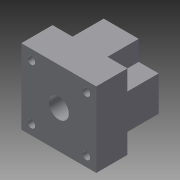
# Autodesk Inventor part: dop_krepl_k_sponke_ne_motora
Saved by Autodesk Inventor 2015 (Build 190159000, 159)
## iProperties
Created: 2016-05-14
Part Number: dop_krepl_k_sponke_ne_motora
Material: Generic
Document SubType Name: Modeling
Designer: Andreas
Density: 1 g/cm^3
Appearance: Default
Author: Andreas
Autodesk Inventor part; units mm, degrees
ref_plane "YZ Plane" through (0, 0, 0) normal (1, 0, 0) x (0, 1, 0)
ref_plane "XZ Plane" through (0, 0, 0) normal (0, 1, 0) x (-1, 0, 0)
ref_plane "XY Plane" through (0, 0, 0) normal (0, 0, 1) x (1, 0, 0)
sketch "Sketch1" plane through (0, 0, 0) normal (0, 1, 0) x (-1, 0, 0)
  line L0 (0, 0) -> (0, -30)
  line L1 (0, -30) -> (30, -30)
  line L2 (30, -30) -> (30, 0)
  line L3 (30, 0) -> (0, 0)
  point P0 (0, -15)
  point P1 (15, 0)
  dimension "d0" = 30
  dimension "d1" = 30
  constraints: 8 end point, 2 midpoint, 2 perpendicular, 1 horizontal, 1 vertical
  measures "d0" distance of L0.start L0.end
  measures "d1" distance of L0.end L1.end
extrude "Extrusion2" add sketch "Sketch1" along normal blind 25
sketch "Sketch5" plane through (0, 25, 0) normal (0, 1, 0) x (1, 0, 0)
  line L0 (0, 0) -> (-8, 0)
  line L1 (-8, 0) -> (-8, 8)
  line L2 (-8, 8) -> (0, 8)
  line L3 (0, 8) -> (0, 0)
  line L4 (0, 30) -> (-8, 30)
  line L5 (-8, 30) -> (-8, 22)
  line L6 (-8, 22) -> (0, 22)
  line L7 (0, 22) -> (0, 30)
  line L8 (-30, 30) -> (-22, 30)
  line L9 (-22, 30) -> (-22, 22)
  line L10 (-22, 22) -> (-30, 22)
  line L11 (-30, 22) -> (-30, 30)
  line L12 (-30, 0) -> (-22, 0)
  line L13 (-22, 0) -> (-22, 8)
  line L14 (-22, 8) -> (-30, 8)
  line L15 (-30, 8) -> (-30, 0)
  dimension "d22" = 8
  dimension "d23" = 8
  dimension "d24" = 8
  dimension "d25" = 8
  dimension "d26" = 8
  dimension "d27" = 8
  dimension "d28" = 8
  dimension "d29" = 8
  constraints: 32 end point, 8 parallel, 4 horizontal, 4 perpendicular
  measures "d22" distance of L1.end L2.end
  measures "d23" distance of L0.end L1.end
  measures "d24" distance of L6.end L5.end
  measures "d25" distance of L5.end L4.end
  measures "d26" distance of L9.end L10.end
  measures "d27" distance of L8.end L9.end
  measures "d28" distance of L14.end L13.end
  measures "d29" distance of L13.end L12.end
extrude "Extrusion6" cut sketch "Sketch5" against normal blind 12.5
sketch "Sketch6" plane through (0, 12.5, 0) normal (0, 1, 0) x (1, 0, 0)
  circle A0 centre (-4, 4) radius 1.5
  circle A1 centre (-26, 4) radius 1.5
  circle A2 centre (-4, 26) radius 1.5
  circle A3 centre (-26, 26) radius 1.5
  point P0 (0, 0)
  dimension "d32" = 3
  dimension "d33" = 3
  dimension "d34" = 3
  dimension "d35" = 3
  constraints: 4 centre point
  measures "d32" diameter of A0
  measures "d33" diameter of A1
  measures "d34" diameter of A2
  measures "d35" diameter of A3
extrude "Extrusion7" cut sketch "Sketch6" against normal up to next
sketch "Sketch7" plane through (0, 0, 0) normal (0, -1, 0) x (1, 0, 0)
  circle A0 centre (-15, -15) radius 4
  point P0 (0, 0)
  dimension "d38" = 8
  constraints: 1 centre point
  measures "d38" diameter of A0
extrude "Extrusion8" cut sketch "Sketch7" against normal blind 20
sketch "Sketch8" plane through (-15, 20, -15) normal (0, -1, 0) x (1, 0, 0)
  circle A0 centre (0, 0) radius 1.5
  point P0 (15, 15)
  dimension "d41" = 3
  constraints: 1 centre point
  measures "d41" diameter of A0
extrude "Extrusion9" cut sketch "Sketch8" against normal up to next
body "Solid2"
